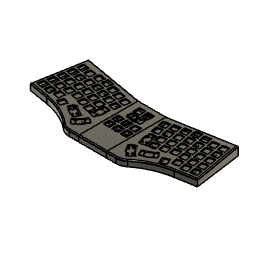
epssp75 case (Autodesk Fusion 360 design; units mm, degrees)
Autodesk Fusion 360 part; units mm, degrees
(part 1 of 3)
sketch "Skizze1" plane through (0, 0, 0) normal (0, 0, 1) x (1, 0, 0)
  line L0 (-114.0111, 89.0308) -> (-100.2238, 86.5997)
  line L1 (-110.3714, 138.7542) -> (-124.1587, 141.1852)
  line L2 (-93.6078, 124.1209) -> (-91.1767, 137.9082)
  line L3 (-111.58, 102.8181) -> (-114.0111, 89.0308)
  line L4 (-94.4847, 119.1476) -> (-108.272, 121.5787)
  line L5 (-97.7927, 100.387) -> (-111.58, 102.8181)
  line L6 (-133.2058, 89.8768) -> (-119.4185, 87.4457)
  line L7 (-124.1587, 141.1852) -> (-126.5898, 127.3979)
  line L8 (-91.1767, 137.9082) -> (-104.964, 140.3393)
  line L9 (-113.6794, 119.9936) -> (-127.4667, 122.4247)
  line L10 (-116.9874, 101.233) -> (-130.7747, 103.6641)
  line L11 (-126.5898, 127.3979) -> (-112.8025, 124.9669)
  line L12 (-100.2238, 86.5997) -> (-97.7927, 100.387)
  line L13 (-107.3951, 126.552) -> (-93.6078, 124.1209)
  line L14 (-119.4185, 87.4457) -> (-116.9874, 101.233)
  line L15 (-112.8025, 124.9669) -> (-110.3714, 138.7542)
  line L16 (-130.7747, 103.6641) -> (-133.2058, 89.8768)
  line L17 (-104.964, 140.3393) -> (-107.3951, 126.552)
  line L18 (-116.1105, 106.2063) -> (-113.6794, 119.9936)
  line L19 (-96.9158, 105.3603) -> (-94.4847, 119.1476)
  line L20 (-108.272, 121.5787) -> (-110.7031, 107.7914)
  line L21 (-129.8978, 108.6374) -> (-116.1105, 106.2063)
  line L22 (-110.7031, 107.7914) -> (-96.9158, 105.3603)
  line L23 (-127.4667, 122.4247) -> (-129.8978, 108.6374)
  line L24 (-120.2954, 82.4724) -> (-134.0827, 84.9035)
  line L25 (-136.5138, 71.1162) -> (-122.7265, 68.6851)
  line L26 (-122.7265, 68.6851) -> (-120.2954, 82.4724)
  line L27 (-134.0827, 84.9035) -> (-136.5138, 71.1162)
  line L28 (-123.6034, 63.7118) -> (-137.3907, 66.1429)
  line L29 (-139.8218, 52.3556) -> (-126.0345, 49.9245)
  line L30 (-126.0345, 49.9245) -> (-123.6034, 63.7118)
  line L31 (-137.3907, 66.1429) -> (-139.8218, 52.3556)
  line L32 (-101.1007, 81.6264) -> (-114.888, 84.0575)
  line L33 (-117.3191, 70.2702) -> (-103.5318, 67.8391)
  line L34 (-103.5318, 67.8391) -> (-101.1007, 81.6264)
  line L35 (-114.888, 84.0575) -> (-117.3191, 70.2702)
  line L36 (-153.6247, 83.7798) -> (-156.0558, 69.9925)
  line L37 (-174.8164, 73.3005) -> (-161.0291, 70.8695)
  line L38 (-164.3371, 52.1089) -> (-161.906, 65.8962)
  line L39 (-150.3167, 102.5404) -> (-152.7478, 88.7531)
  line L40 (-175.6933, 68.3273) -> (-178.1244, 54.5399)
  line L41 (-135.6525, 105.0826) -> (-133.2214, 118.8699)
  line L42 (-154.4131, 108.3906) -> (-151.982, 122.1779)
  line L43 (-178.1244, 54.5399) -> (-164.3371, 52.1089)
  line L44 (-136.5294, 100.1094) -> (-150.3167, 102.5404)
  line L45 (-149.4398, 107.5137) -> (-135.6525, 105.0826)
  line L46 (-156.0558, 69.9925) -> (-142.2685, 67.5615)
  line L47 (-172.3853, 87.0878) -> (-174.8164, 73.3005)
  line L48 (-151.1051, 127.1512) -> (-148.674, 140.9385)
  line L49 (-138.9605, 86.3221) -> (-136.5294, 100.1094)
  line L50 (-133.2214, 118.8699) -> (-147.0087, 121.301)
  line L51 (-161.906, 65.8962) -> (-175.6933, 68.3273)
  line L52 (-143.7007, 140.0616) -> (-146.1318, 126.2743)
  line L53 (-148.674, 140.9385) -> (-162.4613, 143.3696)
  line L54 (-146.1318, 126.2743) -> (-132.3445, 123.8432)
  line L55 (-152.7478, 88.7531) -> (-138.9605, 86.3221)
  line L56 (-168.2004, 110.8217) -> (-154.4131, 108.3906)
  line L57 (-171.5084, 92.0611) -> (-157.7211, 89.6301)
  line L58 (-158.598, 84.6568) -> (-172.3853, 87.0878)
  line L59 (-151.982, 122.1779) -> (-165.7693, 124.609)
  line L60 (-157.7211, 89.6301) -> (-155.29, 103.4174)
  line L61 (-129.9134, 137.6305) -> (-143.7007, 140.0616)
  line L62 (-164.8924, 129.5823) -> (-151.1051, 127.1512)
  line L63 (-165.7693, 124.609) -> (-168.2004, 110.8217)
  line L64 (-147.0087, 121.301) -> (-149.4398, 107.5137)
  line L65 (-162.4613, 143.3696) -> (-164.8924, 129.5823)
  line L66 (-155.29, 103.4174) -> (-169.0773, 105.8484)
  line L67 (-132.3445, 123.8432) -> (-129.9134, 137.6305)
  line L68 (-169.0773, 105.8484) -> (-171.5084, 92.0611)
  line L69 (-142.2685, 67.5615) -> (-139.8374, 81.3488)
  line L70 (-161.0291, 70.8695) -> (-158.598, 84.6568)
  line L71 (-139.8374, 81.3488) -> (-153.6247, 83.7798)
  line L72 (-159.3638, 51.232) -> (-145.5765, 48.8009)
  line L73 (-145.5765, 48.8009) -> (-143.1454, 62.5882)
  line L74 (-156.9327, 65.0193) -> (-159.3638, 51.232)
  line L75 (-143.1454, 62.5882) -> (-156.9327, 65.0193)
  line L76 (-53.119, 105.2534) -> (-55.55, 91.4661)
  line L77 (-38.4547, 107.7956) -> (-36.0237, 121.583)
  line L78 (-39.3317, 102.8224) -> (-53.119, 105.2534)
  line L79 (-55.55, 91.4661) -> (-41.7627, 89.0351)
  line L80 (-52.242, 110.2267) -> (-38.4547, 107.7956)
  line L81 (-76.1582, 113.3776) -> (-89.9455, 115.8087)
  line L82 (-56.868, 113.0733) -> (-54.437, 126.8606)
  line L83 (-57.7449, 108.1) -> (-71.5323, 110.5311)
  line L84 (-68.2243, 129.2916) -> (-70.6553, 115.5043)
  line L85 (-54.437, 126.8606) -> (-68.2243, 129.2916)
  line L86 (-89.9455, 115.8087) -> (-92.3766, 102.0214)
  line L87 (-41.7627, 89.0351) -> (-39.3317, 102.8224)
  line L88 (-78.5893, 99.5903) -> (-76.1582, 113.3776)
  line L89 (-73.9633, 96.7437) -> (-60.176, 94.3127)
  line L90 (-92.3766, 102.0214) -> (-78.5893, 99.5903)
  line L91 (-36.0237, 121.583) -> (-49.811, 124.014)
  line L92 (-79.4662, 94.617) -> (-93.2535, 97.0481)
  line L93 (-70.6553, 115.5043) -> (-56.868, 113.0733)
  line L94 (-75.2813, 118.3509) -> (-72.8502, 132.1382)
  line L95 (-86.6376, 134.5693) -> (-89.0686, 120.7819)
  line L96 (-49.811, 124.014) -> (-52.242, 110.2267)
  line L97 (-71.5323, 110.5311) -> (-73.9633, 96.7437)
  line L98 (-61.0529, 89.3394) -> (-74.8403, 91.7705)
  line L99 (-72.8502, 132.1382) -> (-86.6376, 134.5693)
  line L100 (-89.0686, 120.7819) -> (-75.2813, 118.3509)
  line L101 (-60.176, 94.3127) -> (-57.7449, 108.1)
  line L102 (-93.2535, 97.0481) -> (-95.6846, 83.2608)
  line L103 (-78.1483, 73.0099) -> (-80.5793, 59.2226)
  line L104 (-81.8973, 80.8297) -> (-79.4662, 94.617)
  line L105 (-66.792, 56.7915) -> (-64.3609, 70.5788)
  line L106 (-95.6846, 83.2608) -> (-81.8973, 80.8297)
  line L107 (-63.484, 75.5521) -> (-61.0529, 89.3394)
  line L108 (-85.2053, 62.0691) -> (-82.7742, 75.8564)
  line L109 (-64.3609, 70.5788) -> (-78.1483, 73.0099)
  line L110 (-74.8403, 91.7705) -> (-77.2713, 77.9832)
  line L111 (-77.2713, 77.9832) -> (-63.484, 75.5521)
  line L112 (-80.5793, 59.2226) -> (-66.792, 56.7915)
  line L113 (-96.5615, 78.2875) -> (-98.9926, 64.5002)
  line L114 (-82.7742, 75.8564) -> (-96.5615, 78.2875)
  line L115 (-98.9926, 64.5002) -> (-85.2053, 62.0691)
  line L116 (-50.0847, 84.943) -> (-50.228, 84.1305)
  line L117 (-48.4372, 59.6476) -> (-51.6181, 60.2085)
  line L118 (-53.4524, 76.2964) -> (-58.081, 77.1126)
  line L119 (-61.4229, 56.8348) -> (-61.7225, 55.136)
  line L120 (-52.9335, 52.7486) -> (-52.7903, 53.561)
  line L121 (-48.6574, 76.9995) -> (-45.4765, 76.4386)
  line L122 (-62.6047, 57.0432) -> (-61.4229, 56.8348)
  line L123 (-44.2937, 74.6815) -> (-48.9223, 75.4976)
  line L124 (-56.1483, 61.0073) -> (-60.5503, 61.7835)
  line L125 (-49.6093, 53.0002) -> (-48.4372, 59.6476)
  line L126 (-53.1876, 77.7982) -> (-53.4524, 76.2964)
  line L127 (-46.7247, 60.8942) -> (-44.2937, 74.6815)
  line L128 (-58.4719, 80.4816) -> (-57.2901, 80.2732)
  line L129 (-57.5896, 78.5744) -> (-53.1876, 77.7982)
  line L130 (-60.512, 63.3252) -> (-55.8834, 62.5091)
  line L131 (-52.7903, 53.561) -> (-49.6093, 53.0002)
  line L132 (-51.3533, 61.7103) -> (-46.7247, 60.8942)
  line L133 (-55.533, 54.0446) -> (-55.6762, 53.2322)
  line L134 (-47.4853, 83.6469) -> (-47.3421, 84.4594)
  line L135 (-45.4765, 76.4386) -> (-44.3044, 83.086)
  line L136 (-56.7171, 83.5231) -> (-57.8988, 83.7315)
  line L137 (-44.3044, 83.086) -> (-47.4853, 83.6469)
  line L138 (-47.3421, 84.4594) -> (-50.0847, 84.943)
  line L139 (-60.5503, 61.7835) -> (-60.8499, 60.0847)
  line L140 (-48.9223, 75.4976) -> (-48.6574, 76.9995)
  line L141 (-55.6762, 53.2322) -> (-52.9335, 52.7486)
  line L142 (-58.081, 77.1126) -> (-60.512, 63.3252)
  line L143 (-56.4175, 85.2219) -> (-56.7171, 83.5231)
  line L144 (-61.7225, 55.136) -> (-55.533, 54.0446)
  line L145 (-57.8988, 83.7315) -> (-58.4719, 80.4816)
  line L146 (-51.6181, 60.2085) -> (-51.3533, 61.7103)
  line L147 (-62.0317, 60.2931) -> (-62.6047, 57.0432)
  line L148 (-55.8834, 62.5091) -> (-56.1483, 61.0073)
  line L149 (-60.8499, 60.0847) -> (-62.0317, 60.2931)
  line L150 (-57.2901, 80.2732) -> (-57.5896, 78.5744)
  line L151 (-50.228, 84.1305) -> (-56.4175, 85.2219)
  line L152 (0, 1.75) -> (0, 22.5)
  line L153 (15.275, 92.8) -> (16.1, 92.8)
  line L154 (8.525, 89.57) -> (15.275, 89.57)
  line L155 (13.55, 103.07) -> (10.25, 103.07)
  line L156 (-7, 88.1) -> (7, 88.1)
  line L157 (10.25, 101.87) -> (8.525, 101.87)
  line L158 (16.1, 92.8) -> (16.1, 95.585)
  line L159 (15.275, 101.87) -> (13.55, 101.87)
  line L160 (13.55, 101.87) -> (13.55, 103.07)
  line L161 (16.1, 95.585) -> (15.275, 95.585)
  line L162 (7, 88.1) -> (7, 92.8)
  line L163 (15.275, 95.585) -> (15.275, 101.87)
  line L164 (10.25, 103.07) -> (10.25, 101.87)
  line L165 (8.525, 101.87) -> (8.525, 97.4)
  line L166 (15.275, 89.57) -> (15.275, 92.8)
  line L167 (7, 97.4) -> (7, 102.1)
  line L168 (7, 92.8) -> (8.525, 92.8)
  line L169 (8.525, 92.8) -> (8.525, 89.57)
  line L170 (8.525, 97.4) -> (7, 97.4)
  line L171 (-8.525, 89.57) -> (-8.525, 92.8)
  line L172 (-7, 92.8) -> (-7, 88.1)
  line L173 (-16.1, 95.585) -> (-16.1, 92.8)
  line L174 (-15.275, 92.8) -> (-15.275, 89.57)
  line L175 (-7, 97.4) -> (-8.525, 97.4)
  line L176 (-15.275, 95.585) -> (-16.1, 95.585)
  line L177 (-15.275, 89.57) -> (-8.525, 89.57)
  line L178 (-8.525, 92.8) -> (-7, 92.8)
  line L179 (-10.25, 101.87) -> (-10.25, 103.07)
  line L180 (-13.55, 103.07) -> (-13.55, 101.87)
  line L181 (-8.525, 101.87) -> (-10.25, 101.87)
  line L182 (-13.55, 101.87) -> (-15.275, 101.87)
  line L183 (-15.275, 101.87) -> (-15.275, 95.585)
  line L184 (-8.525, 97.4) -> (-8.525, 101.87)
  line L185 (-10.25, 103.07) -> (-13.55, 103.07)
  line L186 (-7, 102.1) -> (-7, 97.4)
  line L187 (7, 102.1) -> (-7, 102.1)
  line L188 (-16.1, 92.8) -> (-15.275, 92.8)
  line L189 (-2.525, 121.15) -> (-16.525, 121.15)
  line L190 (-16.525, 121.15) -> (-16.525, 107.15)
  line L191 (-16.525, 107.15) -> (-2.525, 107.15)
  line L192 (-2.525, 107.15) -> (-2.525, 121.15)
  line L193 (16.525, 107.15) -> (16.525, 121.15)
  line L194 (2.525, 107.15) -> (16.525, 107.15)
  line L195 (16.525, 121.15) -> (2.525, 121.15)
  line L196 (2.525, 121.15) -> (2.525, 107.15)
  line L197 (7, 83.05) -> (-7, 83.05)
  line L198 (12.05, 83.05) -> (12.05, 69.05)
  line L199 (26.05, 69.05) -> (26.05, 83.05)
  line L200 (-7, 69.05) -> (7, 69.05)
  line L201 (12.05, 69.05) -> (26.05, 69.05)
  line L202 (-7, 83.05) -> (-7, 69.05)
  line L203 (7, 69.05) -> (7, 83.05)
  line L204 (26.05, 83.05) -> (12.05, 83.05)
  line L205 (-12.05, 83.05) -> (-26.05, 83.05)
  line L206 (-12.05, 69.05) -> (-12.05, 83.05)
  line L207 (-26.05, 83.05) -> (-26.05, 69.05)
  line L208 (-26.05, 69.05) -> (-12.05, 69.05)
  line L209 (-26.05, 50) -> (-12.05, 50)
  line L210 (-12.05, 64) -> (-26.05, 64)
  line L211 (-12.05, 50) -> (-12.05, 64)
  line L212 (7, 64) -> (-7, 64)
  line L213 (-26.05, 64) -> (-26.05, 50)
  line L214 (-7, 64) -> (-7, 50)
  line L215 (26.05, 64) -> (12.05, 64)
  line L216 (7, 50) -> (7, 64)
  line L217 (12.05, 50) -> (26.05, 50)
  line L218 (26.05, 50) -> (26.05, 64)
  line L219 (12.05, 64) -> (12.05, 50)
  line L220 (-7, 50) -> (7, 50)
  line L221 (-118.2734, 55.556) -> (-123.0617, 42.4003)
  line L222 (-105.1177, 50.7677) -> (-118.2734, 55.556)
  line L223 (-109.906, 37.6121) -> (-105.1177, 50.7677)
  line L224 (-123.0617, 42.4003) -> (-109.906, 37.6121)
  line L225 (-73.7452, 28.8886) -> (-72.1302, 31.6859)
  line L226 (-72.1302, 31.6859) -> (-71.4157, 31.2734)
  line L227 (-97.1947, 49.3727) -> (-97.9092, 49.7852)
  line L228 (-99.3017, 47.3734) -> (-98.5872, 46.9609)
  line L229 (-94.3566, 40.7886) -> (-92.7416, 43.5859)
  line L230 (-77.9758, 35.0609) -> (-79.5908, 32.2636)
  line L231 (-93.7709, 38.753) -> (-81.6465, 31.753)
  line L232 (-100.2022, 44.1636) -> (-94.3566, 40.7886)
  line L233 (-97.9092, 49.7852) -> (-99.3017, 47.3734)
  line L234 (-70.0232, 33.6852) -> (-70.7377, 34.0977)
  line L235 (-86.7709, 50.8774) -> (-89.1209, 46.8071)
  line L236 (-67.5952, 39.5407) -> (-69.0891, 40.4032)
  line L237 (-69.0891, 40.4032) -> (-68.4891, 41.4424)
  line L238 (-73.4408, 42.9157) -> (-75.6758, 39.0446)
  line L239 (-89.1005, 53.3424) -> (-91.9583, 54.9924)
  line L240 (-91.4209, 42.8234) -> (-93.7709, 38.753)
  line L241 (-90.4416, 47.5696) -> (-88.2066, 51.4407)
  line L242 (-68.4891, 41.4424) -> (-71.3469, 43.0924)
  line L243 (-91.9583, 54.9924) -> (-92.5583, 53.9532)
  line L244 (-89.7005, 52.3032) -> (-89.1005, 53.3424)
  line L245 (-74.6465, 43.8774) -> (-86.7709, 50.8774)
  line L246 (-89.1209, 46.8071) -> (-90.4416, 47.5696)
  line L247 (-98.5872, 46.9609) -> (-100.2022, 44.1636)
  line L248 (-70.7377, 34.0977) -> (-67.5952, 39.5407)
  line L249 (-79.2965, 35.8234) -> (-77.9758, 35.0609)
  line L250 (-92.5583, 53.9532) -> (-94.0522, 54.8157)
  line L251 (-75.6758, 39.0446) -> (-76.9965, 39.8071)
  line L252 (-79.5908, 32.2636) -> (-73.7452, 28.8886)
  line L253 (-88.2066, 51.4407) -> (-89.7005, 52.3032)
  line L254 (-92.7416, 43.5859) -> (-91.4209, 42.8234)
  line L255 (-71.9469, 42.0532) -> (-73.4408, 42.9157)
  line L256 (-71.4157, 31.2734) -> (-70.0232, 33.6852)
  line L257 (-76.9965, 39.8071) -> (-74.6465, 43.8774)
  line L258 (-71.3469, 43.0924) -> (-71.9469, 42.0532)
  line L259 (-94.0522, 54.8157) -> (-97.1947, 49.3727)
  line L260 (-81.6465, 31.753) -> (-79.2965, 35.8234)
  line L261 (-55.409, 39.683) -> (-51.9848, 36.8098)
  line L262 (-45.8408, 29.6636) -> (-49.4412, 32.6847)
  line L263 (-51.9848, 36.8098) -> (-52.965, 35.6416)
  line L264 (-51.0702, 44.8538) -> (-52.179, 43.5324)
  line L265 (-46.2556, 40.8139) -> (-51.0702, 44.8538)
  line L266 (-54.3002, 41.0045) -> (-55.409, 39.683)
  line L267 (-52.179, 43.5324) -> (-53.0982, 44.3037)
  line L268 (-43.5918, 39.6557) -> (-45.7253, 41.4459)
  line L269 (-45.9866, 31.7767) -> (-41.6478, 36.9475)
  line L270 (-41.6478, 36.9475) -> (-44.1221, 39.0237)
  line L271 (-49.4412, 32.6847) -> (-48.461, 33.8529)
  line L272 (-55.2194, 41.7758) -> (-54.3002, 41.0045)
  line L273 (-48.461, 33.8529) -> (-45.9866, 31.7767)
  line L274 (-66.3685, 26.622) -> (-67.4773, 25.3005)
  line L275 (-58.4402, 21.9601) -> (-54.8398, 18.939)
  line L276 (-69.5985, 22.7726) -> (-70.7073, 21.4512)
  line L277 (-67.4773, 25.3005) -> (-68.3966, 26.0719)
  line L278 (-70.7073, 21.4512) -> (-65.8927, 17.4113)
  line L279 (-65.8927, 17.4113) -> (-66.423, 16.7793)
  line L280 (-62.9443, 23.7487) -> (-66.3685, 26.622)
  line L281 (-65.5644, 27.938) -> (-61.964, 24.9169)
  line L282 (-66.423, 16.7793) -> (-64.2896, 14.9891)
  line L283 (-68.3966, 26.0719) -> (-70.5178, 23.5439)
  line L284 (-61.285, 13.5449) -> (-56.9462, 18.7157)
  line L285 (-63.7593, 15.6211) -> (-61.285, 13.5449)
  line L286 (-56.9462, 18.7157) -> (-59.4205, 20.7919)
  line L287 (-59.4205, 20.7919) -> (-58.4402, 21.9601)
  line L288 (-70.5178, 23.5439) -> (-69.5985, 22.7726)
  line L289 (-56.5654, 38.6627) -> (-65.5644, 27.938)
  line L290 (-54.8398, 18.939) -> (-45.8408, 29.6636)
  line L291 (-61.964, 24.9169) -> (-62.9443, 23.7487)
  line L292 (-64.2896, 14.9891) -> (-63.7593, 15.6211)
  line L293 (-52.965, 35.6416) -> (-56.5654, 38.6627)
  line L294 (-45.7253, 41.4459) -> (-46.2556, 40.8139)
  line L295 (-53.0982, 44.3037) -> (-55.2194, 41.7758)
  line L296 (-44.1221, 39.0237) -> (-43.5918, 39.6557)
  line L297 (-120.1528, 56.2401) -> (-124.9411, 43.0844) construction
  line L298 (-103.2383, 50.0837) -> (-108.0266, 36.928) construction
  line L299 (-118.2734, 55.556) -> (-109.906, 37.6121) construction
  line L300 (-105.1177, 50.7677) -> (-123.0617, 42.4003) construction
  line L301 (-86.7709, 50.8774) -> (-81.6465, 31.753) construction
  line L302 (-74.6465, 43.8774) -> (-93.7709, 38.753) construction
  line L303 (-114.0897, 46.584) -> (-84.2087, 41.3152) construction
  line L304 (-67.0965, 29.2236) -> (-72.4156, 22.8846) construction
  line L305 (-44.7551, 60.5469) -> (-46.7607, 49.1723) construction
  line L306 (-46.7607, 49.1723) -> (-53.359, 50.3358) construction
  line L307 (-58.0975, 39.9482) -> (-50.6733, 48.796) construction
  line L308 (-50.6733, 48.796) -> (-48.965, 47.3626) construction
  line L309 (-166.5386, 157.8222) -> (-33.7619, 134.4101)
  line L310 (-166.5386, 157.8222) -> (-185.963, 47.6611)
  line L311 (-185.963, 47.6611) -> (-142.0159, 39.9121)
  arc A0 (-71.1177, 6.8517) -> (-142.0159, 39.9121) centre (-168.2583, -108.916) ccw
  line L312 (-71.1177, 6.8517) -> (-47.1498, -13.2597) construction
  line L313 (1.75, 0) -> (22.5, 0)
  line L314 (-31.075, 0) -> (-31.075, 134.175)
  line L315 (31.075, 0) -> (31.075, 134.175)
  line L316 (-31.075, 0) -> (31.075, 0)
  line L317 (31.075, 134.175) -> (-31.075, 134.175)
  arc A1 (-33.7619, 134.4101) -> (-31.075, 134.175) centre (-31.075, 149.6482) ccw
  arc A2 (-71.1177, 6.8517) -> (-52.2928, 0) centre (-52.2928, 29.2863) ccw
  line L318 (-52.2928, 0) -> (-31.075, 0)
  line L319 (-125.2934, 36.2688) -> (-112.1377, 31.4806) construction
  line L320 (12.05, 69.05) -> (7, 64) construction
  line L321 (-7, 69.05) -> (-12.05, 64) construction
  circle A3 centre (9.525, 66.525) radius 1.25
  circle A4 centre (9.525, 66.525) radius 2.25
  circle A5 centre (-9.525, 66.525) radius 1.25
  circle A6 centre (-9.525, 66.525) radius 2.25
  circle A7 centre (-19.05, 104.625) radius 1.25
  circle A8 centre (-19.05, 104.625) radius 2.25
  circle A9 centre (19.05, 104.625) radius 1.25
  circle A10 centre (19.05, 104.625) radius 2.25
  circle A11 centre (-21.525, 28.425) radius 1.25
  circle A12 centre (-21.525, 28.425) radius 2.25
  circle A13 centre (21.525, 28.425) radius 1.25
  circle A14 centre (21.525, 28.425) radius 2.25
  line L322 (21.525, 28.425) -> (-21.525, 28.425) construction
  line L323 (-156.9327, 65.0193) -> (-161.0291, 70.8695) construction
  line L324 (-151.5323, 95.6468) -> (-156.5055, 96.5237) construction
  line L325 (-151.1051, 127.1512) -> (-147.0087, 121.301) construction
  circle A15 centre (-149.0569, 124.2261) radius 1.25
  circle A16 centre (-149.0569, 124.2261) radius 2.25
  circle A17 centre (-154.0189, 96.0852) radius 1.25
  circle A18 centre (-154.0189, 96.0852) radius 2.25
  circle A19 centre (-158.9809, 67.9444) radius 1.25
  circle A20 centre (-158.9809, 67.9444) radius 2.25
  line L326 (-57.7449, 108.1) -> (-52.242, 110.2267) construction
  line L327 (-63.484, 75.5521) -> (-64.3609, 70.5788) construction
  circle A21 centre (-63.9225, 73.0654) radius 1.25
  circle A22 centre (-63.9225, 73.0654) radius 2.25
  circle A23 centre (-54.9935, 109.1633) radius 1.25
  circle A24 centre (-54.9935, 109.1633) radius 2.25
  circle A25 centre (-61.9903, 41.0135) radius 1.25
  circle A26 centre (-61.9903, 41.0135) radius 2.25
  line L328 (-89.0686, 120.7819) -> (-94.4847, 119.1476) construction
  line L329 (-108.272, 121.5787) -> (-112.8025, 124.9669) construction
  line L330 (-118.203, 94.3393) -> (-112.7956, 95.9244) construction
  line L331 (-99.0082, 93.4934) -> (-94.4691, 90.1544) construction
  line L332 (-117.3191, 70.2702) -> (-118.6301, 62.8349) construction
  line L333 (-118.6301, 62.8349) -> (-123.6034, 63.7118) construction
  circle A27 centre (-121.1168, 63.2734) radius 1.25
  circle A28 centre (-121.1168, 63.2734) radius 2.25
  circle A29 centre (-99, 55) radius 1.25
  circle A30 centre (-99, 55) radius 2.25
  circle A31 centre (-96.7387, 91.8239) radius 1.25
  circle A32 centre (-96.7387, 91.8239) radius 2.25
  circle A33 centre (-115.4993, 95.1319) radius 1.25
  circle A34 centre (-115.4993, 95.1319) radius 2.25
  circle A35 centre (-91.7767, 119.9648) radius 1.25
  circle A36 centre (-91.7767, 119.9648) radius 2.25
  circle A37 centre (-110.5373, 123.2728) radius 1.25
  circle A38 centre (-110.5373, 123.2728) radius 2.25
  line L334 (-16.525, 107.15) -> (-21.575, 102.1) construction
  line L335 (16.525, 107.15) -> (21.575, 102.1) construction
  circle A39 centre (19.05, 104.625) radius 1
  circle A40 centre (-19.05, 104.625) radius 1
  circle A41 centre (-9.525, 66.525) radius 1
  circle A42 centre (9.525, 66.525) radius 1
  circle A43 centre (21.525, 28.425) radius 1
  circle A44 centre (-21.525, 28.425) radius 1
  circle A45 centre (-54.9935, 109.1633) radius 1
  circle A46 centre (-91.7767, 119.9648) radius 1
  circle A47 centre (-110.5373, 123.2728) radius 1
  circle A48 centre (-149.0569, 124.2261) radius 1
  circle A49 centre (-154.0189, 96.0852) radius 1
  circle A50 centre (-115.4993, 95.1319) radius 1
  circle A51 centre (-96.7387, 91.8239) radius 1
  circle A52 centre (-63.9225, 73.0654) radius 1
  circle A53 centre (-158.9809, 67.9444) radius 1
  circle A54 centre (-121.1168, 63.2734) radius 1
  circle A55 centre (-99, 55) radius 1
  circle A56 centre (-61.9903, 41.0135) radius 1
  circle A57 centre (-9.525, 66.525) radius 3.5
  circle A58 centre (9.525, 66.525) radius 3.5
  circle A59 centre (-21.525, 28.425) radius 3.5
  circle A60 centre (21.525, 28.425) radius 3.5
  circle A61 centre (19.05, 104.625) radius 3.5
  circle A62 centre (-19.05, 104.625) radius 3.5
  point P0 (0, 88.1)
  point P1 (-120.6676, 48.9782)
  point P2 (-124.4122, 47.6076)
  point P3 (-114.0897, 46.584)
  point P4 (-84.2087, 41.3152)
  point P5 (-104.7735, 42.796)
  point P6 (-72.6439, 24.246)
  point P7 (-31.075, 120.7104)
  dimension "d2" = 14
  dimension "d3" = 14
  dimension "d6" = 14
  dimension "d7" = 14
  dimension "d9" = 14
  dimension "d10" = 14
  dimension "d11" = 14
  dimension "d12" = 14
  dimension "d13" = 5.05
  dimension "d14" = 14
  dimension "d15" = 14
  dimension "d16" = 14
  dimension "d17" = 14
  dimension "d128" = 14
  dimension "d129" = 14
  dimension "d130" = 14
  dimension "d131" = 14
  dimension "d132" = 5.05
  dimension "d133" = 5.05
  dimension "d134" = 5.05
  dimension "d135" = 5.05
  dimension "d136" = 5.05
  dimension "d137" = 5.05
  dimension "d138" = 14
  dimension "d139" = 14
  dimension "d140" = 5.05
  dimension "d141" = 2.5
  dimension "d142" = 14
  dimension "d143" = 14
  dimension "d144" = 14
  dimension "d145" = 14
  dimension "d146" = 14
  dimension "d147" = 14
  dimension "d148" = 14
  dimension "d149" = 14
  dimension "d150" = 5.05
  dimension "d151" = 14
  dimension "d152" = 14
  dimension "d153" = 14
  dimension "d154" = 14
  dimension "d155" = 14
  dimension "d156" = 14
  dimension "d157" = 14
  dimension "d158" = 14
  dimension "d159" = 5.05
  dimension "d160" = 5.05
  dimension "d161" = 5.05
  dimension "d162" = 5.05
  dimension "d163" = 5.05
  dimension "d164" = 5.05
  dimension "d165" = 14
  dimension "d166" = 14
  dimension "d167" = 5.05
  dimension "d169" = 5.05
  dimension "d170" = 14
  dimension "d171" = 14
  dimension "d172" = 5.05
  dimension "d173" = 7
  dimension "d176" = 14
  dimension "d177" = 14
  dimension "d180" = 14
  dimension "d181" = 14
  dimension "d191" = 5.05
  dimension "d201" = 14
  dimension "d202" = 14
  dimension "d203" = 14
  dimension "d204" = 14
  dimension "d205" = 14
  dimension "d206" = 14
  dimension "d207" = 14
  dimension "d208" = 14
  dimension "d209" = 5.05
  dimension "d210" = 14
  dimension "d211" = 14
  dimension "d212" = 14
  dimension "d213" = 14
  dimension "d214" = 14
  dimension "d215" = 14
  dimension "d218" = 5.05
  dimension "d219" = 5.05
  dimension "d220" = 5.05
  dimension "d221" = 5.05
  dimension "d222" = 5.05
  dimension "d224" = 14
  dimension "d225" = 14
  dimension "d226" = 5.05
  dimension "d227" = 5.05
  dimension "d232" = 5.05
  dimension "d234" = 4.5
  dimension "d235" = 6.5
  dimension "d236" = 3.3
  dimension "d237" = 1.2
  dimension "d238" = 1.725
  dimension "d239" = 1.725
  dimension "d240" = 1.725
  dimension "d241" = 1.725
  dimension "d242" = 3.3
  dimension "d245" = 6.75
  dimension "d246" = 6.75
  dimension "d247" = 3.23
  dimension "d248" = 4.7
  dimension "d249" = 14
  dimension "d250" = 14
  dimension "d251" = 6.285
  dimension "d252" = 0.825
  dimension "d254" = 2.785
  dimension "d255" = 1.525
  dimension "d256" = 4.47
  dimension "d257" = 4.7
  dimension "d258" = 14.575
  dimension "d261" = 3.3
  dimension "d262" = 1.2
  dimension "d263" = 1.725
  dimension "d264" = 1.725
  dimension "d265" = 1.725
  dimension "d266" = 1.725
  dimension "d267" = 3.3
  dimension "d268" = 6.75
  dimension "d269" = 6.75
  dimension "d270" = 3.23
  dimension "d271" = 4.7
  dimension "d272" = 14
  dimension "d273" = 14
  dimension "d274" = 6.285
  dimension "d275" = 0.825
  dimension "d276" = 2.785
  dimension "d277" = 1.525
  dimension "d278" = 4.47
  dimension "d279" = 4.7
  dimension "d280" = 14
  dimension "d281" = 14
  dimension "d282" = 14
  dimension "d283" = 14
  dimension "d284" = 5.05
  dimension "d285" = 5.05
  dimension "d286" = 2.525
  dimension "d287" = 14
  dimension "d288" = 14
  dimension "d289" = 14
  dimension "d290" = 14
  dimension "d291" = 5.05
  dimension "d292" = 14
  dimension "d293" = 14
  dimension "d294" = 5.05
  dimension "d295" = 14
  dimension "d296" = 14
  dimension "d297" = 14
  dimension "d298" = 14
  dimension "d300" = 14
  dimension "d301" = 14
  dimension "d303" = 5.05
  dimension "d305" = 5.05
  dimension "d306" = 14
  dimension "d307" = 14
  dimension "d312" = 3.3
  dimension "d313" = 1.2
  dimension "d314" = 1.725
  dimension "d315" = 1.725
  dimension "d316" = 1.725
  dimension "d317" = 1.725
  dimension "d318" = 3.3
  dimension "d319" = 6.75
  dimension "d320" = 6.75
  dimension "d321" = 3.23
  dimension "d322" = 4.7
  dimension "d323" = 14
  dimension "d324" = 14
  dimension "d325" = 6.285
  dimension "d326" = 0.825
  dimension "d327" = 2.785
  dimension "d328" = 1.525
  dimension "d329" = 4.47
  dimension "d330" = 4.7
  dimension "d375" = 3.3
  dimension "d376" = 1.2
  dimension "d377" = 1.725
  dimension "d378" = 1.725
  dimension "d379" = 1.725
  dimension "d380" = 1.725
  dimension "d381" = 3.3
  dimension "d382" = 6.75
  dimension "d383" = 6.75
  dimension "d384" = 3.23
  dimension "d385" = 4.7
  dimension "d386" = 14
  dimension "d387" = 14
  dimension "d388" = 6.285
  dimension "d389" = 0.825
  dimension "d390" = 2.785
  dimension "d391" = 1.525
  dimension "d392" = 4.47
  dimension "d393" = 4.7
  dimension "d395" = 50
  dimension "d399" = 10
  dimension "d401" = 2
  dimension "d402" = 2
  dimension "d403" = 2
  dimension "d404" = 1.05
  dimension "d405" = 2
  dimension "d407" = 10
  dimension "d408" = 2
  dimension "d409" = 11.55
  dimension "d410" = 1.05
  dimension "d411" = 2
  dimension "d412" = 11.55
  dimension "d413" = 2
  dimension "d414" = 1.05
  dimension "d415" = 2
  dimension "d416" = 11.55
  dimension "d418" = 10
  dimension "d419" = 2
  dimension "d420" = 11.55
  dimension "d421" = 1.05
  dimension "d423" = 6.525
  dimension "d424" = 6.525
  dimension "d494" = 10
  dimension "d496" = 5.025
  dimension "d497" = 5.025
  dimension "d498" = 5.025
  dimension "d499" = 13.025
  dimension "d512" = 6.525
  dimension "d543" = 2.5
  dimension "d544" = 4.5
  dimension "d545" = 2.5
  dimension "d546" = 4.5
  dimension "d547" = 2.5
  dimension "d548" = 4.5
  dimension "d550" = 2.5
  dimension "d551" = 4.5
  dimension "d553" = 2.5
  dimension "d554" = 4.5
  dimension "d555" = 2.5
  dimension "d556" = 4.5
  dimension "d557" = 9.55
  dimension "d558" = 9.55
  dimension "d587" = 2.5
  dimension "d588" = 4.5
  dimension "d589" = 2.5
  dimension "d590" = 4.5
  dimension "d591" = 2.5
  dimension "d592" = 4.5
  dimension "d593" = 2.5
  dimension "d594" = 4.5
  dimension "d595" = 2.5
  dimension "d596" = 4.5
  dimension "d597" = 2.5
  dimension "d598" = 4.5
  dimension "d599" = 2.5
  dimension "d600" = 4.5
  dimension "d601" = 2.5
  dimension "d602" = 4.5
  dimension "d603" = 2.5
  dimension "d604" = 4.5
  dimension "d605" = 2.5
  dimension "d606" = 4.5
  dimension "d607" = 2.5
  dimension "d608" = 4.5
  dimension "d609" = 2.5
  dimension "d610" = 4.5
  dimension "d611" = 170
  dimension "d617" = 135
  dimension "d618" = 135
  dimension "d620" = 38.1
  dimension "d621" = 38.1
  dimension "d645" = 2
  dimension "d649" = 2
  dimension "d651" = 2
  dimension "d653" = 2
  dimension "d655" = 2
  dimension "d657" = 2
  dimension "d661" = 2
  dimension "d662" = 2
  dimension "d663" = 2
  dimension "d664" = 2
  dimension "d665" = 2
  dimension "d666" = 2
  dimension "d667" = 2
  dimension "d668" = 2
  dimension "d669" = 2
  dimension "d670" = 2
  dimension "d671" = 2
  dimension "d672" = 2
  dimension "d705" = 7
  dimension "d706" = 7
  dimension "d707" = 7
  dimension "d708" = 7
  dimension "d709" = 7
  dimension "d710" = 7
  constraint perpendicular L4 L20
  constraint perpendicular L20 L22
  constraint perpendicular L9 L23
  constraint perpendicular L21 L23
  constraint perpendicular L8 L17
  constraint perpendicular L13 L17
  constraint perpendicular L1 L7
  constraint perpendicular L7 L11
  constraint collinear L15 L18
  constraint collinear L2 L19
  constraint perpendicular L3 L5
  constraint perpendicular L0 L3
  constraint perpendicular L10 L16
  constraint perpendicular L6 L16
  constraint collinear L14 L18
  constraint collinear L12 L19
  constraint perpendicular L24 L27
  constraint perpendicular L25 L27
  constraint perpendicular L28 L31
  constraint perpendicular L29 L31
  constraint perpendicular L32 L35
  constraint perpendicular L33 L35
  constraint collinear L14 L26
  constraint collinear L26 L30
  constraint collinear L12 L34
  constraint perpendicular L2 L8
  constraint perpendicular L1 L15
  constraint perpendicular L50 L64
  constraint perpendicular L45 L64
  constraint perpendicular L59 L63
  constraint perpendicular L56 L63
  constraint perpendicular L52 L61
  constraint perpendicular L52 L54
  constraint perpendicular L53 L65
  constraint perpendicular L62 L65
  constraint collinear L42 L48
  constraint collinear L41 L67
  constraint perpendicular L39 L44
  constraint perpendicular L39 L55
  constraint perpendicular L66 L68
  constraint perpendicular L57 L68
  constraint collinear L42 L60
  constraint collinear L41 L49
  constraint perpendicular L47 L58
  constraint perpendicular L37 L47
  constraint perpendicular L40 L51
  constraint perpendicular L40 L43
  constraint perpendicular L36 L71
  constraint perpendicular L36 L46
  constraint collinear L60 L70
  constraint collinear L38 L70
  constraint collinear L49 L69
  constraint perpendicular L61 L67
  constraint perpendicular L48 L53
  constraint perpendicular L74 L75
  constraint perpendicular L72 L74
  constraint collinear L69 L73
  constraint collinear L53 L61
  constraint perpendicular L76 L78
  constraint perpendicular L76 L79
  constraint perpendicular L91 L96
  constraint perpendicular L80 L96
  constraint collinear L77 L87
  constraint perpendicular L77 L91
  constraint perpendicular L83 L97
  constraint perpendicular L89 L97
  constraint perpendicular L81 L86
  constraint perpendicular L86 L90
  constraint perpendicular L84 L85
  constraint perpendicular L84 L93
  constraint perpendicular L95 L99
  constraint perpendicular L95 L100
  constraint collinear L88 L94
  constraint collinear L82 L101
  constraint perpendicular L98 L110
  constraint perpendicular L110 L111
  constraint perpendicular L92 L102
  constraint perpendicular L102 L106
  constraint collinear L88 L104
  constraint collinear L101 L107
  constraint perpendicular L113 L114
  constraint perpendicular L113 L115
  constraint perpendicular L103 L109
  constraint perpendicular L103 L112
  constraint collinear L104 L108
  constraint collinear L105 L107
  constraint perpendicular L82 L85
  constraint perpendicular L94 L99
  constraint collinear L1 L99
  constraint perpendicular L143 L151
  constraint perpendicular L116 L151
  constraint perpendicular L116 L138
  constraint perpendicular L134 L138
  constraint perpendicular L134 L137
  constraint perpendicular L135 L137
  constraint perpendicular L121 L135
  constraint perpendicular L121 L140
  constraint perpendicular L123 L140
  constraint perpendicular L123 L127
  constraint perpendicular L127 L132
  constraint perpendicular L132 L146
  constraint perpendicular L117 L146
  constraint perpendicular L117 L125
  constraint perpendicular L125 L131
  constraint perpendicular L120 L131
  constraint perpendicular L120 L141
  constraint perpendicular L133 L141
  constraint perpendicular L133 L144
  constraint perpendicular L119 L144
  constraint perpendicular L119 L122
  constraint perpendicular L122 L147
  constraint perpendicular L147 L149
  constraint perpendicular L139 L149
  constraint perpendicular L124 L139
  constraint perpendicular L124 L148
  constraint perpendicular L130 L148
  constraint perpendicular L130 L142
  constraint perpendicular L118 L142
  constraint perpendicular L118 L126
  constraint perpendicular L126 L129
  constraint perpendicular L129 L150
  constraint perpendicular L128 L150
  constraint perpendicular L128 L145
  constraint perpendicular L136 L145
  constraint collinear L137 L151
  constraint collinear L131 L144
  constraint collinear L121 L129
  constraint collinear L118 L123
  constraint collinear L130 L132
  constraint collinear L117 L124
  constraint collinear L125 L135
  constraint collinear L119 L139
  constraint collinear L139 L150
  constraint collinear L143 L150
  constraint collinear L145 L147
  constraint collinear L140 L146
  constraint collinear L126 L148
  constraint collinear L120 L146
  constraint collinear L134 L140
  constraint collinear L116 L133
  constraint equal L116 L133
  constraint equal L140 L146
  constraint parallel L79 L151
  constraint collinear L87 L127
  constraint perpendicular L159 L163
  constraint perpendicular L161 L163
  constraint perpendicular L158 L161
  constraint perpendicular L153 L158
  constraint perpendicular L153 L166
  constraint perpendicular L154 L166
  constraint perpendicular L154 L169
  constraint perpendicular L168 L169
  constraint perpendicular L162 L168
  constraint perpendicular L156 L162
  constraint perpendicular L156 L172
  constraint perpendicular L172 L178
  constraint perpendicular L171 L178
  constraint perpendicular L171 L177
  constraint perpendicular L174 L177
  constraint perpendicular L174 L188
  constraint perpendicular L173 L188
  constraint perpendicular L173 L176
  constraint perpendicular L176 L183
  constraint perpendicular L182 L183
  constraint perpendicular L180 L182
  constraint perpendicular L180 L185
  constraint perpendicular L179 L185
  constraint perpendicular L179 L181
  constraint perpendicular L181 L184
  constraint perpendicular L175 L184
  constraint perpendicular L175 L186
  constraint perpendicular L186 L187
  constraint perpendicular L167 L187
  constraint perpendicular L167 L170
  constraint perpendicular L165 L170
  constraint perpendicular L157 L165
  constraint perpendicular L157 L164
  constraint perpendicular L155 L164
  constraint perpendicular L155 L160
  constraint collinear L163 L166
  constraint collinear L174 L183
  constraint collinear L165 L169
  constraint collinear L162 L167
  constraint collinear L172 L186
  constraint collinear L171 L184
  constraint collinear L154 L177
  constraint collinear L181 L182
  constraint collinear L157 L181
  constraint collinear L157 L159
  constraint collinear L155 L185
  constraint collinear L168 L178
  constraint collinear L170 L175
  constraint collinear L178 L188
  constraint collinear L153 L168
  constraint collinear L161 L176
  constraint equal L161 L176
  constraint equal L168 L178
  constraint midpoint L156 P0
  constraint coincident L152 P0
  constraint perpendicular L189 L190
  constraint perpendicular L190 L191
  constraint perpendicular L189 L192
  constraint perpendicular L195 L196
  constraint perpendicular L194 L196
  constraint perpendicular L193 L195
  constraint collinear L189 L195
  constraint horizontal L156
  constraint perpendicular L197 L202
  constraint perpendicular L200 L202
  constraint perpendicular L197 L203
  constraint perpendicular L198 L204
  constraint perpendicular L198 L201
  constraint perpendicular L199 L204
  constraint collinear L197 L204
  constraint perpendicular L205 L207
  constraint perpendicular L207 L208
  constraint perpendicular L205 L206
  constraint collinear L197 L205
  constraint perpendicular L212 L214
  constraint perpendicular L214 L220
  constraint perpendicular L212 L216
  constraint perpendicular L215 L219
  constraint perpendicular L217 L219
  constraint perpendicular L215 L218
  constraint collinear L212 L215
  constraint perpendicular L210 L213
  constraint perpendicular L209 L213
  constraint perpendicular L210 L211
  constraint collinear L210 L212
  constraint collinear L206 L211
  constraint collinear L198 L219
  constraint collinear L202 L214
  constraint collinear L172 L202
  constraint perpendicular L221 L222
  constraint perpendicular L221 L224
  constraint perpendicular L222 L223
  constraint perpendicular L236 L248
  constraint perpendicular L234 L248
  constraint perpendicular L234 L256
  constraint perpendicular L226 L256
  constraint perpendicular L225 L226
  constraint perpendicular L225 L252
  constraint perpendicular L230 L252
  constraint perpendicular L230 L249
  constraint perpendicular L249 L260
  constraint perpendicular L231 L260
  constraint perpendicular L231 L240
  constraint perpendicular L240 L254
  constraint perpendicular L229 L254
  constraint perpendicular L229 L232
  constraint perpendicular L232 L247
  constraint perpendicular L228 L247
  constraint perpendicular L228 L233
  constraint perpendicular L227 L233
  constraint perpendicular L227 L259
  constraint perpendicular L250 L259
  constraint perpendicular L243 L250
  constraint perpendicular L239 L243
  constraint perpendicular L239 L244
  constraint perpendicular L244 L253
  constraint perpendicular L241 L253
  constraint perpendicular L241 L246
  constraint perpendicular L235 L246
  constraint perpendicular L235 L245
  constraint perpendicular L245 L257
  constraint perpendicular L251 L257
  constraint perpendicular L238 L251
  constraint perpendicular L238 L255
  constraint perpendicular L255 L258
  constraint perpendicular L242 L258
  constraint perpendicular L237 L242
  constraint collinear L225 L248
  constraint collinear L247 L259
  constraint collinear L230 L238
  constraint collinear L257 L260
  constraint collinear L235 L240
  constraint collinear L229 L241
  constraint collinear L232 L252
  constraint collinear L250 L253
  constraint collinear L253 L255
  constraint collinear L236 L255
  constraint collinear L239 L242
  constraint collinear L249 L254
  constraint collinear L246 L251
  constraint collinear L228 L254
  constraint collinear L226 L249
  constraint collinear L227 L234
  constraint equal L227 L234
  constraint equal L249 L254
  constraint perpendicular L264 L265
  constraint perpendicular L265 L294
  constraint perpendicular L268 L294
  constraint perpendicular L268 L296
  constraint perpendicular L270 L296
  constraint perpendicular L269 L270
  constraint perpendicular L269 L273
  constraint perpendicular L271 L273
  constraint perpendicular L262 L271
  constraint perpendicular L262 L290
  constraint perpendicular L275 L290
  constraint perpendicular L275 L287
  constraint perpendicular L286 L287
  constraint perpendicular L284 L286
  constraint perpendicular L284 L285
  constraint perpendicular L285 L292
  constraint perpendicular L282 L292
  constraint perpendicular L279 L282
  constraint perpendicular L278 L279
  constraint perpendicular L276 L278
  constraint perpendicular L276 L288
  constraint perpendicular L283 L288
  constraint perpendicular L277 L283
  constraint perpendicular L274 L277
  constraint perpendicular L274 L280
  constraint perpendicular L280 L291
  constraint perpendicular L281 L291
  constraint perpendicular L281 L289
  constraint perpendicular L289 L293
  constraint perpendicular L263 L293
  constraint perpendicular L261 L263
  constraint perpendicular L261 L266
  constraint perpendicular L266 L272
  constraint perpendicular L272 L295
  constraint perpendicular L267 L295
  constraint collinear L265 L270
  constraint collinear L278 L285
  constraint collinear L261 L273
  constraint collinear L262 L293
  constraint collinear L275 L281
  constraint collinear L280 L286
  constraint collinear L269 L284
  constraint collinear L274 L276
  constraint collinear L266 L274
  constraint collinear L264 L266
  constraint collinear L283 L295
  constraint collinear L271 L287
  constraint collinear L263 L291
  constraint collinear L287 L292
  constraint collinear L271 L296
  constraint collinear L279 L294
  constraint equal L279 L294
  constraint equal L271 L287
  constraint midpoint L221 P1
  constraint coincident L29 P1
  constraint perpendicular L222 L297
  constraint coincident L222 L297.start
  constraint coincident L224 L297.end
  constraint coincident L222 L298.start
  constraint coincident L224 L298.end
  constraint perpendicular L222 L298
  constraint midpoint L300 P3
  constraint midpoint L302 P4
  constraint coincident P3 L303.start
  constraint coincident P4 L303.end
  constraint parallel L115 L303
  constraint parallel L289 L304
  constraint coincident L281 L304.start
  constraint perpendicular L117 L305
  constraint perpendicular L146 L306
  constraint coincident L132 L305.start
  constraint coincident L120 L306.end
  constraint perpendicular L272 L307
  constraint perpendicular L289 L308
  constraint coincident L293 L307.start
  constraint coincident L264 L308.end
  constraint coincident L278 L304.end
  constraint parallel L8 L309
  constraint perpendicular L309 L310
  constraint perpendicular L310 L311
  constraint tangent L311 A0
  constraint tangent A0 L312
  constraint parallel L285 L312
  constraint coincident L31 L311.end
  constraint coincident L77 L309.end
  constraint vertical L314
  constraint coincident L314 P7
  constraint coincident L91 P7
  constraint perpendicular L314 L317
  constraint tangent L317 A1
  constraint tangent L309 A1
  constraint tangent A0 A2
  constraint perpendicular L314 L318
  constraint tangent A2 L318
  constraint collinear L313 L316
  constraint parallel L224 L319
  constraint coincident L221 L319.start
  constraint coincident L223 L319.end
  constraint tangent A0 L319
  constraint coincident L287 A0.start
  constraint midpoint L320 A3.centre
  constraint concentric A3 A4
  constraint midpoint L321 A5.centre
  constraint concentric A5 A6
  constraint concentric A7 A8
  constraint concentric A9 A10
  constraint concentric A11 A12
  constraint concentric A13 A14
  constraint coincident A13.centre A14.centre
  constraint coincident A11.centre A12.centre
  constraint horizontal L322
  constraint midpoint L39 L324.start
  constraint midpoint L60 L324.end
  constraint midpoint L325 A15.centre
  constraint concentric A15 A16
  constraint midpoint L324 A17.centre
  constraint concentric A17 A18
  constraint midpoint L323 A19.centre
  constraint concentric A19 A20
  constraint midpoint L327 A21.centre
  constraint concentric A21 A22
  constraint midpoint L326 A23.centre
  constraint concentric A23 A24
  constraint concentric A25 A26
  constraint midpoint L14 L330.start
  constraint midpoint L3 L330.end
  constraint midpoint L12 L331.start
  constraint midpoint L102 L331.end
  constraint collinear L28 L333
  constraint collinear L35 L332
  constraint midpoint L333 A27.centre
  constraint concentric A27 A28
  constraint concentric A29 A30
  constraint midpoint L331 A31.centre
  constraint concentric A31 A32
  constraint midpoint L330 A33.centre
  constraint concentric A33 A34
  constraint midpoint L328 A35.centre
  constraint concentric A35 A36
  constraint midpoint L329 A37.centre
  constraint concentric A37 A38
  constraint equal L325 L334
  constraint midpoint A7.centre L334
  constraint equal L334 L335
  constraint midpoint A9.centre L335
  constraint concentric A9 A39
  constraint concentric A7 A40
  constraint concentric A5 A41
  constraint concentric A3 A42
  constraint concentric A14 A43
  constraint concentric A12 A44
  constraint concentric A23 A45
  constraint concentric A35 A46
  constraint concentric A38 A47
  constraint concentric A16 A48
  constraint concentric A17 A49
  constraint concentric A34 A50
  constraint concentric A31 A51
  constraint concentric A22 A52
  constraint concentric A19 A53
  constraint concentric A28 A54
  constraint concentric A29 A55
  constraint concentric A25 A56
  constraint concentric A6 A57
  constraint concentric A3 A58
  constraint concentric A11 A59
  constraint concentric A13 A60
  constraint concentric A9 A61
  constraint concentric A7 A62
  measures "d2" distance of L4.start L4.end
  measures "d3" distance of L20.end L4.end
  measures "d6" distance of L9.end L21.start
  measures "d7" distance of L18.start L21.start
  measures "d9" distance of L13.start L8.end
  measures "d10" distance of L13.start L2.start
  measures "d11" distance of L7.end L1.end
  measures "d12" distance of L7.end L11.end
  measures "d13" distance of L15 L17
  measures "d14" distance of L3.start L0.start
  measures "d15" distance of L0.end L0.start
  measures "d16" distance of L6.start L10.end
  measures "d17" distance of L6.start L6.end
  measures "d128" distance of L25.start L24.end
  measures "d129" distance of L25.start L25.end
  measures "d130" distance of L29.start L28.end
  measures "d131" distance of L29.start L29.end
  measures "d132" distance of L9 L11
  measures "d133" distance of L4 L13
  measures "d134" distance of L10 L21
  measures "d135" distance of L5 L22
  measures "d136" distance of L6 L24
  measures "d137" distance of L25 L28
  measures "d138" distance of L33.start L32.end
  measures "d139" distance of L33.start L33.end
  measures "d140" distance of L0 L32
  measures "d141" distance of L1 L8
  measures "d142" distance of L50.end L41.end
  measures "d143" distance of L50.end L45.start
  measures "d144" distance of L56.start L59.end
  measures "d145" distance of L42.start L56.start
  measures "d146" distance of L52.start L52.end
  measures "d147" distance of L52.end L54.end
  measures "d148" distance of L53.end L62.start
  measures "d149" distance of L48.start L62.start
  measures "d150" distance of L48 L52
  measures "d151" distance of L39.start L39.end
  measures "d152" distance of L49.start L39.end
  measures "d153" distance of L57.start L66.end
  measures "d154" distance of L57.start L57.end
  measures "d155" distance of L47.start L37.start
  measures "d156" distance of L37.end L37.start
  measures "d157" distance of L40.end L40.start
  measures "d158" distance of L40.end L38.start
  measures "d159" distance of L59 L62
  measures "d160" distance of L50 L54
  measures "d161" distance of L56 L66
  measures "d162" distance of L44 L45
  measures "d163" distance of L57 L58
  measures "d164" distance of L37 L51
  measures "d165" distance of L36.end L36.start
  measures "d166" distance of L36.end L46.end
  measures "d167" distance of L55 L71
  measures "d169" distance of L7 L67
  measures "d170" distance of L72.start L74.start
  measures "d171" distance of L72.start L72.end
  measures "d172" distance of L46 L75
  measures "d173" distance of L8 L61
  measures "d176" distance of L76.end L76.start
  measures "d177" distance of L79.end L76.end
  measures "d180" distance of L91.end L80.start
  measures "d181" distance of L77.start L80.start
  measures "d191" distance of L78 L80
  measures "d201" distance of L83.start L83.end
  measures "d202" distance of L89.start L83.end
  measures "d203" distance of L86.end L81.end
  measures "d204" distance of L88.start L86.end
  measures "d205" distance of L84.start L84.end
  measures "d206" distance of L82.start L84.end
  measures "d207" distance of L95.end L95.start
  measures "d208" distance of L95.end L94.start
  measures "d209" distance of L84 L94
  measures "d210" distance of L110.end L98.end
  measures "d211" distance of L107.start L110.end
  measures "d212" distance of L102.end L92.end
  measures "d213" distance of L102.end L104.start
  measures "d214" distance of L113.start L113.end
  measures "d215" distance of L108.start L113.end
  measures "d218" distance of L81 L100
  measures "d219" distance of L83 L93
  measures "d220" distance of L90 L92
  measures "d221" distance of L89 L98
  measures "d222" distance of L106 L114
  measures "d224" distance of L103.start L103.end
  measures "d225" distance of L103.end L105.start
  measures "d226" distance of L109 L111
  measures "d227" distance of L82 L96
  measures "d232" distance of L2 L95
  measures "d234" distance of L8 L85
  measures "d235" distance of L8 L91
  measures "d236" distance of L136.end L128.start
  measures "d237" distance of L136.start L136.end
  measures "d238" distance of L136.start L143.start
  measures "d239" distance of L129.start L128.end
  measures "d240" distance of L124.end L139.end
  measures "d241" distance of L119.end L119.start
  measures "d242" distance of L147.start L122.start
  measures "d245" distance of L135.end L121.end
  measures "d246" distance of L117.start L125.start
  measures "d247" distance of L134.start L135.end
  measures "d248" distance of L123.end L123.start
  measures "d249" distance of L127.start L123.start
  measures "d250" distance of L127 L142
  measures "d251" distance of L116.end L143.start
  measures "d252" distance of L138 L151
  measures "d254" distance of L116.start L134.end
  measures "d255" distance of L121.start L123.end
  measures "d256" distance of L129.start L126.start
  measures "d257" distance of L118.end L118.start
  measures "d258" distance of L79 L123
  measures "d261" distance of L155.end L155.start
  measures "d262" distance of L159.end L155.start
  measures "d263" distance of L159.end L159.start